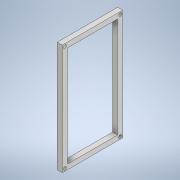
# Autodesk Inventor part: Cadre encoche manette
Saved by Autodesk Inventor 2021 (Build 250183000, 183)
## iProperties
Created: 2020-09-19
Part Number: Cadre encoche manette
Material: Générique
Document SubType Name: Modeling
Designer: Utilisateur
Density: 1 g/cm^3
Appearance: Par défaut
Author: Utilisateur
Autodesk Inventor part; units mm, degrees
ref_plane "YZ Plane" through (0, 0, 0) normal (1, 0, 0) x (0, 1, 0)
ref_plane "XZ Plane" through (0, 0, 0) normal (0, 1, 0) x (-1, 0, 0)
ref_plane "XY Plane" through (0, 0, 0) normal (0, 0, 1) x (1, 0, 0)
sketch "Esquisse1" plane through (0, 0, 0) normal (1, 0, 0) x (0, 1, 0)
  line L0 (10, 5) -> (-10, 5)
  line L1 (-10, 5) -> (-10, -5)
  line L2 (-10, -5) -> (10, -5)
  line L3 (10, -5) -> (10, 5)
  line L4 (10, 5) -> (-10, -5) construction
  line L5 (-10, 5) -> (10, -5) construction
  line L6 (11, 6) -> (-11, 6)
  line L7 (-11, 6) -> (-11, -6)
  line L8 (-11, -6) -> (11, -6)
  line L9 (11, -6) -> (11, 6)
  line L10 (11, 6) -> (-11, -6) construction
  line L11 (-11, 6) -> (11, -6) construction
  line L12 (-11, 6) -> (-10, 5) construction
  circle A0 centre (-10.5, 5.5) radius 0.3042
  line L13 (-10, -5) -> (-11, -6) construction
  circle A1 centre (-10.5, -5.5) radius 0.3042
  line L14 (0, 12.1344) -> (0, -11.0693) construction
  line L15 (0, -11.0693) -> (0, -10.4091)
  line L16 (10, 5) -> (11, 6) construction
  line L17 (10, -5) -> (11, -6) construction
  circle A2 centre (10.5, 5.5) radius 0.3042
  circle A3 centre (10.5, -5.5) radius 0.3042
  point P0 (0, 0)
  point P1 (0, 0)
  point P2 (0, 0)
  dimension "d0" = 10
  dimension "d1" = 20
  dimension "d2" = 22
  dimension "d3" = 12
  dimension "d4" = 0.6083
  dimension "d5" = 0.6083
  dimension "d6" = 0.6083
  dimension "d7" = 0.6083
  constraints: 36 end point, 9 midpoint, 4 centre point, 4 parallel, 2 horizontal, 2 perpendicular
  measures "d0" distance of L2.end L0.start
  measures "d1" distance of L0.start L0.end
  measures "d2" distance of L6.start L6.end
  measures "d3" distance of L6.end L7.end
  measures "d4" diameter of A0
  measures "d5" diameter of A1
  measures "d6" diameter of A2
  measures "d7" diameter of A3
extrude "Extrusion1" add sketch "Esquisse1" along normal blind 1
